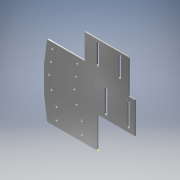
# Autodesk Inventor part: base_plate
Saved by Autodesk Inventor 2018 (Build 220112000, 112)
## iProperties
Created: 2018-04-04
Part Number: base_plate
Material: アルミニウム 6061
Document SubType Name: モデリング
Designer: NaMACHAN
Density: 2.7 g/cm^3
Appearance: アルミニウム - フラット
Sheet Metal Rule: Default
Author: NaMACHAN
Autodesk Inventor part; units mm, degrees
ref_plane "YZ Plane" through (0, 0, 0) normal (1, 0, 0) x (0, 1, 0)
ref_plane "XZ Plane" through (0, 0, 0) normal (0, 1, 0) x (-1, 0, 0)
ref_plane "XY Plane" through (0, 0, 0) normal (0, 0, 1) x (1, 0, 0)
sketch "スケッチ1" plane through (0, 0, 0) normal (0, 1, 0) x (-1, 0, 0)
  line L0 (0, 0) -> (80, 0)
  line L1 (80, 0) -> (85, 38)
  line L2 (85, 38) -> (85, 76)
  line L3 (85, 76) -> (80, 114)
  line L4 (-50, 100) -> (-50, 154)
  line L5 (0, 0) -> (0, 50)
  line L6 (-60, 50) -> (-60, 100)
  line L7 (-60, 100) -> (-50, 100)
  line L8 (0, 50) -> (-60, 50)
  line L9 (80, 114) -> (20, 114)
  line L10 (20, 114) -> (20, 154)
  line L11 (20, 154) -> (-50, 154)
  dimension "d4" = 38
  dimension "d6" = 5
  dimension "d29" = 80
  dimension "d34" = 38
  dimension "d128" = 38
  dimension "d182" = 50
  dimension "d186" = 50
  dimension "d190" = 40
  dimension "d192" = 70
  dimension "d203" = 60
  dimension "d204" = 60
  constraints: 25 end point, 6 perpendicular, 3 horizontal, 1 coincident, 1 vertical, 1 vertical alignment
  measures "d4" vertical distance of L0.end L1.end
  measures "d6" horizontal distance of L0.end L1.end
  measures "d29" distance of L0.start L0.end
  measures "d34" vertical distance of L3.end L2.end
  measures "d128" distance of L1.end L2.end
  measures "d182" distance of L0.start L5.end
  measures "d186" distance of L6.start L6.end
  measures "d190" distance of L9.end L10.end
  measures "d192" distance of L10.end L4.end
  measures "d203" distance of L3.end L9.end
  measures "d204" distance of L5.end L6.start
extrude "押し出し1" add sketch "スケッチ1" along normal blind 2
fillet "フィレット1" radius 2 4 edges at (50, 1, 154) (-80, 1, 114) (0, 1, 0) (-80, 1, 0)
sketch "スケッチ8" plane through (0, 2, 0) normal (0, 1, 0) x (1, 0, 0)
  point P0 (0, 0)
  point P1 (-65, -9.5)
  point P2 (-25, -9.5)
  point P3 (-25, -28.5)
  point P4 (-65, -28.5)
  point P5 (-73, -47.5)
  point P6 (-33, -47.5)
  point P7 (-77, -66.5)
  point P8 (-37, -66.5)
  point P9 (-34, -85.5)
  point P10 (-74, -85.5)
  point P11 (-72, -104.5)
  point P12 (-32, -104.5)
  dimension "d132" = 40
  dimension "d133" = 40
  dimension "d134" = 40
  dimension "d135" = 40
  dimension "d136" = 40
  dimension "d137" = 40
  dimension "d138" = 9.5
  dimension "d139" = 25
  dimension "d141" = 19
  dimension "d143" = 19
  dimension "d144" = 19
  dimension "d145" = 19
  dimension "d146" = 19
  dimension "d147" = 8
  dimension "d148" = 4
  dimension "d149" = 3
  dimension "d150" = 2
  constraints: 6 horizontal alignment, 1 vertical alignment
  measures "d132" distance of point (-25, -9.5) point (-65, -9.5)
  measures "d133" distance of point (-65, -28.5) point (-25, -28.5)
  measures "d134" distance of point (-73, -47.5) point (-33, -47.5)
  measures "d135" distance of point (-77, -66.5) point (-37, -66.5)
  measures "d136" distance of point (-34, -85.5) point (-74, -85.5)
  measures "d137" distance of point (-32, -104.5) point (-72, -104.5)
  measures "d138" vertical distance of point (0, 0) point (-25, -9.5)
  measures "d139" horizontal distance of point (0, 0) point (-25, -9.5)
  measures "d141" distance of point (-25, -28.5) point (-25, -9.5)
  measures "d143" vertical distance of point (-33, -47.5) point (-25, -28.5)
  measures "d144" vertical distance of point (-37, -66.5) point (-33, -47.5)
  measures "d145" vertical distance of point (-34, -85.5) point (-37, -66.5)
  measures "d146" vertical distance of point (-32, -104.5) point (-34, -85.5)
  measures "d147" horizontal distance of point (-25, -28.5) point (-33, -47.5)
  measures "d148" horizontal distance of point (-37, -66.5) point (-33, -47.5)
  measures "d149" horizontal distance of point (-34, -85.5) point (-37, -66.5)
  measures "d150" horizontal distance of point (-34, -85.5) point (-32, -104.5)
hole "穴6" at (-65, 2, 9.5) at (-25, 2, 9.5) at (-25, 2, 28.5) at (-65, 2, 28.5) at (-73, 2, 47.5) at (-33, 2, 47.5) at (-77, 2, 66.5) at (-37, 2, 66.5) at (-34, 2, 85.5) at (-74, 2, 85.5) at (-72, 2, 104.5) at (-32, 2, 104.5) direction (0, -1, 0) diameter 3 end through all
sketch "スケッチ11" plane through (0, 2, 0) normal (0, 1, 0) x (1, 0, 0)
  line L0 (38, -114) -> (38, -149)
  arc A0 (34, -149) -> (38, -149) centre (36, -149) ccw
  line L1 (34, -149) -> (34, -114)
  arc A1 (38, -114) -> (34, -114) centre (36, -114) ccw
  line L2 (-20, -154) -> (48, -154) projected
  line L3 (50, -152) -> (50, -100) projected
  line L4 (8, -114) -> (8, -149)
  arc A2 (4, -149) -> (8, -149) centre (6, -149) ccw
  line L5 (4, -149) -> (4, -114)
  arc A3 (8, -114) -> (4, -114) centre (6, -114) ccw
  point P0 (0, 0)
  dimension "d194" = 2
  dimension "d195" = 5
  dimension "d196" = 12
  dimension "d197" = 40
  dimension "d198" = 2
  dimension "d199" = 30
  constraints: 8 end point, 8 point on circle, 8 tangent, 4 centre point, 2 horizontal alignment, 2 parallel, 2 vertical
  measures "d194" radius of A1
  measures "d195" distance from line of L2 A0.centre
  measures "d196" distance between parallel lines of L3 L0
  measures "d197" distance from line of L2 A1.centre
  measures "d198" radius of A2
  measures "d199" distance of A0.centre A2.centre
extrude "押し出し3" cut sketch "スケッチ11" against normal blind 10
sketch "スケッチ12" plane through (0, 2, 0) normal (0, 1, 0) x (1, 0, 0)
  point P0 (0, 0)
sketch "スケッチ13" plane through (0, 2, 0) normal (0, 1, 0) x (1, 0, 0)
  line L0 (48, -92) -> (48, -58)
  arc A0 (52, -58) -> (48, -58) centre (50, -58) ccw
  line L1 (52, -58) -> (52, -92)
  arc A1 (48, -92) -> (52, -92) centre (50, -92) ccw
  line L2 (16, -92) -> (16, -58)
  arc A2 (16, -58) -> (12, -58) centre (14, -58) ccw
  line L3 (12, -58) -> (12, -92)
  arc A3 (12, -92) -> (16, -92) centre (14, -92) ccw
  line L4 (60, -100) -> (60, -50) projected
  line L5 (50, -100) -> (60, -100) projected
  line L6 (60, -50) -> (0, -50) projected
  point P0 (0, 0)
  dimension "d205" = 2
  dimension "d206" = 2
  dimension "d207" = 10
  dimension "d208" = 8
  dimension "d209" = 8
  dimension "d210" = 36
  constraints: 8 end point, 8 point on circle, 8 tangent, 4 centre point, 2 horizontal alignment, 2 parallel, 2 vertical
  measures "d205" radius of A3
  measures "d206" radius of A1
  measures "d207" distance from line of L4 A1.centre
  measures "d208" distance from line of L5 A1.centre
  measures "d209" distance from line of L6 A0.centre
  measures "d210" distance of A0.centre A2.centre
extrude "押し出し4" cut sketch "スケッチ13" against normal blind 10
